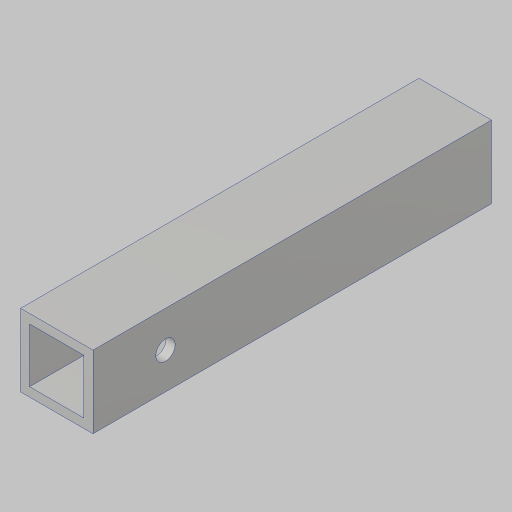
# Autodesk Inventor part: CHD-003
Saved by Autodesk Inventor 2023.5 (Build 275446000, 446)
## iProperties
Created: 2025-02-02
Part Number: CHD-003
Material: Aluminum 6061
Document SubType Name: Modeling
Designer: slick
Mass: 304.185 g
Surface Area: 718.547 cm^2
Volume: 112.661 cm^3
Density: 2.7 g/cm^3
Appearance: Aluminum - Flat
RuleStatus: InUse
AfterDocNew0: SHOW
AfterDocOpen0: SHOW
Author: slick
Autodesk Inventor part; units mm, degrees
ref_plane "YZ Plane" through (0, 0, 0) normal (1, 0, 0) x (0, 1, 0)
ref_plane "XZ Plane" through (0, 0, 0) normal (0, 1, 0) x (-1, 0, 0)
ref_plane "XY Plane" through (0, 0, 0) normal (0, 0, 1) x (1, 0, 0)
sketch "Sketch1" plane through (0, 0, 0) normal (0, 0, 1) x (1, 0, 0)
  line L0 (-12.7, -12.7) -> (12.7, -12.7)
  line L1 (12.7, -12.7) -> (12.7, 12.7)
  line L2 (12.7, 12.7) -> (-12.7, 12.7)
  line L3 (-12.7, 12.7) -> (-12.7, -12.7)
  line L4 (-12.7, -12.7) -> (12.7, 12.7) construction
  line L5 (12.7, -12.7) -> (-12.7, 12.7) construction
  line L6 (-9.525, 9.525) -> (9.525, 9.525)
  line L7 (9.525, 9.525) -> (9.525, -9.525)
  line L8 (9.525, -9.525) -> (-9.525, -9.525)
  line L9 (-9.525, -9.525) -> (-9.525, 9.525)
  point P0 (0, 0)
  dimension "width" = 25.4
  dimension "height" = 25.4
  dimension "thickness" = 3.175
  constraints: 20 end point, 4 parallel, 2 midpoint, 2 perpendicular, 1 horizontal, 3 other
  measures "width" distance of L2.end L1.end
  measures "height" distance of L1.end L0.end
  measures "thickness" distance between parallel lines of L2 L6
extrude "Extrusion1" add sketch "Sketch1" along normal mid plane 139.7
sketch "Sketch2" plane through (12.7, -12.7, 69.85) normal (1, 0, 0) x (0, 0, -1)
  line L0 (0, 0) -> (0, 25.4) construction
  point P0 (69.85, 12.7)
  point P1 (25.4, 12.7)
  dimension "d5" = 25.4
  constraints: 1 horizontal alignment
  measures "d5" distance from line of L0 point (25.4, 12.7)
hole "Hole1" at (12.7, 0, 44.45) direction (-1, 0, 0) diameter 6.7564 end through all clearance for "Flat Head Machine Screw (82)" size "1/4" standard "Ansi Unified Screw Threads"
body "Solid1"
